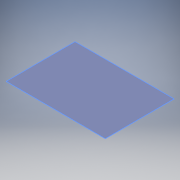
# Autodesk Inventor part: BrennerBrennTeil
Saved by Autodesk Inventor 2018 (Build 220112000, 112)
## iProperties
Created: 2017-11-12
Part Number: BrennerBrennTeil
Material: Titan
Document SubType Name: Modeling
Density: 4.51 g/cm^3
Appearance: Titan
Autodesk Inventor part; units mm, degrees
ref_plane "YZ Plane" through (0, 0, 0) normal (1, 0, 0) x (0, 1, 0)
ref_plane "XZ Plane" through (0, 0, 0) normal (0, 1, 0) x (-1, 0, 0)
ref_plane "XY Plane" through (0, 0, 0) normal (0, 0, 1) x (1, 0, 0)
sketch "Skizze1" plane through (0, 0, 0) normal (0, 0, 1) x (1, 0, 0)
  line L0 (-90, -62.5) -> (-90, 62.5) construction
  line L1 (-90, 62.5) -> (90, 62.5) construction
  line L2 (90, 62.5) -> (90, -62.5) construction
  line L3 (90, -62.5) -> (-90, -62.5) construction
  line L4 (-90, 62.5) -> (90, 62.5)
  line L5 (90, 62.5) -> (90, -62.5)
  line L6 (90, -62.5) -> (-90, -62.5)
  line L7 (-90, -62.5) -> (-90, 62.5)
  point P0 (0, 0)
  constraints: 8 end point, 2 parallel, 1 horizontal, 1 perpendicular
extrude "Extrusion1" add sketch "Skizze1" along normal blind 0.01
